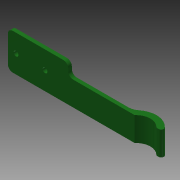
# Autodesk Inventor part: hand2
Saved by Autodesk Inventor 2013 (Build 170138000, 138)
## iProperties
Created: 2014-06-28
Part Number: hand2
Material: Generic
Document SubType Name: Modeling
Designer: Masta
Density: 1 g/cm^3
Author: Masta
Autodesk Inventor part; units mm, degrees
ref_plane "YZ Plane" through (0, 0, 0) normal (1, 0, 0) x (0, 1, 0)
ref_plane "XZ Plane" through (0, 0, 0) normal (0, 1, 0) x (-1, 0, 0)
ref_plane "XY Plane" through (0, 0, 0) normal (0, 0, 1) x (1, 0, 0)
sketch "Sketch1" plane through (0, 0, 0) normal (0, 0, 1) x (1, 0, 0)
  line L0 (0, 0) -> (52.5, 0)
  line L1 (63.5, 0) -> (63.5, 1.5)
  line L2 (0, 1.5) -> (0, 0)
  arc A0 (63.5, 1.5) -> (50.5, 1.5) centre (57, -3.9686) ccw
  arc A1 (61.5, 0) -> (52.5, 0) centre (57, -3.9686) ccw
  line L3 (61.5, 0) -> (63.5, 0)
  line L4 (52.5, 0) -> (61.5, 0) construction
  line L5 (59.4686, 1.5) -> (54.5314, 1.5) construction
  line L6 (54.5314, 1.5) -> (50.5, 1.5) construction
  line L7 (50.5, 1.5) -> (0, 1.5)
  line L8 (63.5, 1.5) -> (59.4686, 1.5) construction
  dimension "d0" = 63.5
  dimension "d1" = 1.5
  dimension "d3" = 9
  dimension "d4" = 6
  dimension "d5" = 2
  constraints: 18 end point, 13 parallel, 6 point on circle, 3 horizontal, 3 perpendicular, 2 centre point, 1 coincident, 1 point on line
  measures "d0" distance of L2.start L1.end
  measures "d1" distance of L1.end L1.start
  measures "d3" distance of L3.start L0.end
  measures "d4" radius of A1
  measures "d5" distance of L1.start L3.start
extrude "Extrusion1" add sketch "Sketch1" along normal blind 15
sketch "Sketch2" plane through (0, 1.5, 0) normal (0, 1, 0) x (1, 0, 0)
  line L0 (50.5, 0) -> (0, 0) projected
  line L1 (0, 0) -> (0, -15) projected
  line L2 (50.5, -15) -> (0, -15) projected
  line L3 (3.38, 0) -> (3.38, -15) construction
  line L4 (3.38, -7.5) -> (15.38, -7.5) construction
  dimension "d9" = 3.38
  dimension "d10" = 12
  constraints: 4 end point, 2 perpendicular, 2 point on line, 1 midpoint
  measures "d9" distance between parallel lines of L3 L1
  measures "d10" distance of L4.start L4.end
hole "Hole1" at (3.38, 1.5, 7.5) at (15.38, 1.5, 7.5) direction (0, -1, 0) diameter 2 end through all
fillet "Fillet1" radius 1 3 edges at (63.5, 0, 7.5) (63.5, 1.5, 7.5) (61.5, 0, 7.5)
fillet "Fillet2" radius 5 1 edges at (50.5, 1.5, 7.5)
sketch "Sketch3" plane through (0, 0, 0) normal (0, -1, 0) x (1, 0, 0)
  line L0 (0, 15) -> (52.5, 15) projected
  line L1 (0, 0) -> (0, 15) projected
  line L2 (25, 20.9607) -> (67.8053, 20.9607)
  line L3 (67.8053, 20.9607) -> (67.8053, 10)
  line L4 (67.8053, 10) -> (25, 10)
  line L5 (25, 10) -> (25, 20.9607)
  dimension "d20" = 5
  dimension "d21" = 25
  constraints: 8 end point, 2 parallel, 1 horizontal, 1 perpendicular
  measures "d20" distance between parallel lines of L4 L0
  measures "d21" distance between parallel lines of L1 L5
extrude "Extrusion2" cut sketch "Sketch3" against normal blind 8
fillet "Fillet3" radius 2 4 edges at (25, 0.75, 15) (25, 0.75, 10) (0, 0.75, 15) (0, 0.75, 0)
body "Solid1"
